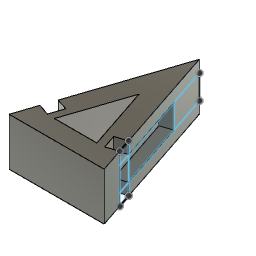
support v2 (Autodesk Fusion 360 design; units mm, degrees)
Autodesk Fusion 360 part; units mm, degrees
sketch "Sketch1" plane through (0, 0, 0) normal (0, 0, 1) x (1, 0, 0)
  line L0 (-10, 0) -> (10, 0)
  line L1 (10, 0) -> (0, 30)
  line L2 (0, 30) -> (-10, 0)
  constraint horizontal L0
extrude "Extrude1" add sketch "Sketch1" along normal blind 10 thin wall 4 inside
sketch "Sketch3" plane through (9, 3, 0) normal (0.948683, 0.316228, 0) x (-0.316228, 0.948683, 0)
  line L0 (-3.1623, 0) -> (28.4605, 0)
  line L1 (28.4605, 0) -> (28.4605, 10)
  line L2 (28.4605, 10) -> (-3.1623, 10)
  line L3 (-3.1623, 10) -> (-3.1623, 0)
  line L4 (28.4605, 7.5013) -> (28.4605, 2.4485)
  line L5 (2, 10) -> (2, 0)
  line L6 (2, 10) -> (5, 10)
  line L7 (5, 0) -> (2, 0)
  line L8 (5, 10) -> (5, 0)
  line L9 (5, 10) -> (2, 10)
  line L10 (5, 0) -> (2, 0)
  line L11 (28.4605, 7.5013) -> (2, 7.5013)
  line L12 (28.4605, 2.4485) -> (2, 2.4485)
  line L13 (20.0146, 7.5013) -> (20.0146, 2.4485)
  constraint coincident L1 L4.start
  constraint coincident L1 L4.end
  constraint coincident L2 L5.start
  constraint coincident L0 L5.end
  constraint perpendicular L0 L5
  constraint coincident L2 L6.end
  constraint coincident L0 L7.start
  constraint perpendicular L7 L8
  constraint coincident L5 L11.end
  constraint perpendicular L5 L11
  constraint coincident L5 L12.end
  constraint coincident L11 L13.start
  constraint coincident L12 L13.end
  constraint perpendicular L12 L13
extrude "Extrude5" cut sketch "Sketch3" against normal blind 2.5 contours L0 L5 L7 L8 L10 L12 | L5 L8 L11 L12 | L2 L5 L6 L8 L9 L11 | L8 L11 L12 L13
sketch "Sketch7" plane through (-9, 3, 0) normal (-0.948683, 0.316228, 0) x (-0.316228, -0.948683, 0)
  line L0 (-28.4605, 0) -> (3.1623, 0)
  line L1 (3.1623, 0) -> (3.1623, 10)
  line L2 (3.1623, 10) -> (-28.4605, 10)
  line L3 (-28.4605, 10) -> (-28.4605, 0)
  line L4 (-1.9689, 10) -> (-1.9689, 0)
  line L5 (-5.0001, 10) -> (-5.0001, 0)
  line L6 (-5.0001, 10) -> (-1.9689, 10)
  line L7 (-5.0001, 0) -> (-1.9689, 0)
  line L8 (-1.9689, 7.4726) -> (-28.4605, 7.4726)
  line L9 (-1.9689, 2.3994) -> (-28.4605, 2.3994)
  line L10 (-28.4605, 7.4726) -> (-28.4605, 2.3994)
  line L11 (-20.0189, 7.4726) -> (-20.0189, 2.3994)
  constraint coincident L2 L4.start
  constraint coincident L0 L4.end
  constraint perpendicular L0 L4
  constraint coincident L2 L5.start
  constraint coincident L0 L5.end
  constraint perpendicular L0 L5
  constraint coincident L4 L8.start
  constraint coincident L3 L8.end
  constraint perpendicular L3 L8
  constraint coincident L4 L9.start
  constraint coincident L3 L9.end
  constraint perpendicular L3 L9
  constraint coincident L8 L11.start
  constraint coincident L9 L11.end
  constraint perpendicular L9 L11
extrude "Extrude6" cut sketch "Sketch7" against normal blind 2.5 contours L0 L4 L5 L7 L9 | L5 L8 L9 L11 | L4 L5 L8 L9 | L2 L4 L5 L6 L8
